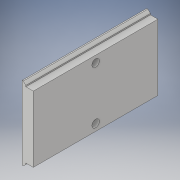
# Autodesk Inventor part: batteryholder9
Saved by Autodesk Inventor 2017 (Build 210142000, 142)
## iProperties
Created: 2020-11-06
Part Number: batteryholder9
Material: Generic
Document SubType Name: Modeling
Designer: agustin
Density: 1 g/cm^3
Appearance: Default
Author: agustin
## iProperties of the stored document batter-holder_3DPrint.ipt
Created: 2021-01-25
Part Number: batter-holder_3DPrint
Material: Generic
Document SubType Name: Modeling
Designer: agustin
Density: 1 g/cm^3
Appearance: Default
Author: agustin
Autodesk Inventor part; units mm, degrees
ref_plane "YZ Plane" through (0, 0, 0) normal (1, 0, 0) x (0, 1, 0)
ref_plane "XZ Plane" through (0, 0, 0) normal (0, 1, 0) x (-1, 0, 0)
ref_plane "XY Plane" through (0, 0, 0) normal (0, 0, 1) x (1, 0, 0)
sketch "Sketch1" plane through (0, 0, 0) normal (0, 0, 1) x (1, 0, 0)
  line L0 (-19.2766, 29.5) -> (-19.2766, -29.4652) projected
  line L1 (-18.2766, -29.4652) -> (-19.2766, -29.4652) projected
  line L2 (-16.2766, -27.4652) -> (-18.2766, -29.4652) projected
  line L3 (-16.2766, -26.5) -> (-16.2766, -27.4652) projected
  line L4 (-16.2766, -26.5) -> (28.7234, -26.5) construction
  arc A0 (28.7234, -26.5) -> (30.7234, -24.5) centre (28.7234, -24.5) ccw projected
  line L5 (30.7234, -24.5) -> (30.7234, -19.5) projected
  line L6 (30.7234, -19.5) -> (27.7234, -22.5) projected
  line L7 (27.7234, -22.5) -> (-14.2766, -22.5) construction
  arc A1 (-16.2766, -20.5) -> (-14.2766, -22.5) centre (-14.2766, -20.5) ccw construction
  line L8 (-16.2766, -20.5) -> (-16.2766, 20.5) construction
  arc A2 (-14.2766, 22.5) -> (-16.2766, 20.5) centre (-14.2766, 20.5) ccw construction
  line L9 (-14.2766, 22.5) -> (27.7234, 22.5) construction
  line L10 (27.7234, 22.5) -> (30.7234, 19.5) projected
  line L11 (30.7234, 19.5) -> (30.7234, 24.5) projected
  arc A3 (30.7234, 24.5) -> (28.7234, 26.5) centre (28.7234, 24.5) ccw projected
  line L12 (28.7234, 26.5) -> (-16.2766, 26.5) construction
  line L13 (-16.2766, 26.5) -> (-16.2766, 27.5) projected
  line L14 (-16.2766, 27.5) -> (-18.2766, 29.5) projected
  line L15 (-18.2766, 29.5) -> (-19.2766, 29.5) projected
  line L16 (-16.2766, -26.5) -> (-10.2766, -26.5)
  line L17 (-10.2766, -26.5) -> (-10.2766, 26.5)
  line L18 (-10.2766, 26.5) -> (-16.2766, 26.5)
  line L19 (-10.2766, 26.5) -> (-16.2766, 26.5)
  line L20 (-19.2766, -29.4652) -> (-19.2766, 29.5)
  line L21 (-18.2766, 29.5) -> (-19.2766, 29.5)
  line L22 (-18.2766, 29.5) -> (-16.2766, 27.5)
  line L23 (-16.2766, 27.5) -> (-16.2766, 26.5)
  line L24 (-19.2766, -29.4652) -> (-18.2766, -29.4652)
  line L25 (-18.2766, -29.4652) -> (-16.2766, -27.4652)
  line L26 (-16.2766, -27.4652) -> (-16.2766, -26.5)
  point P0 (0, 0)
  dimension "d0" = 6
  constraints: 22 end point, 6 collinear, 3 perpendicular, 2 point on circle, 1 horizontal, 1 parallel, 1 point on line
  measures "d0" distance of L18.end L17.end
extrude "Extrusion1" add sketch "Sketch1" along normal blind 100
sketch "Sketch2" plane through (-10.2766, -26.5, 0) normal (1, 0, 0) x (0, 0, -1)
  line L0 (0, -2.9652) -> (0, -0.9652) projected
  line L1 (-100, 56) -> (-100, -2.9652) projected
  line L2 (0, -2.9652) -> (-100, -2.9652) projected
  line L3 (-100, 56) -> (-100, -2.9652)
  line L4 (0, 56) -> (0, -2.9652) projected
  line L5 (0, 56) -> (-100, 56) projected
  circle A0 centre (-50, 5.5174) radius 3
  circle A1 centre (-50, 47.5174) radius 3
  point P0 (0, 26.5)
  dimension "d5" = 6
  dimension "d6" = 6
  constraints: 2 centre point, 2 end point, 1 perpendicular
  measures "d5" diameter of A0
  measures "d6" diameter of A1
extrude "Extrusion2" cut sketch "Sketch2" against normal blind 100 contours A0 | A1
scale "Scale1" factors (0.5, 0.5, 0.5) then translate (-9.6383, 0.0087, 25) bodies 1
body "Solid1"
